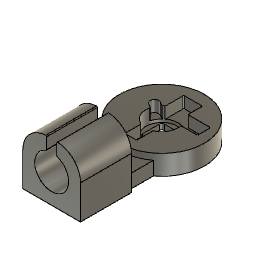
miniscope holder niko's version v13 (Autodesk Fusion 360 design; units mm, degrees)
Autodesk Fusion 360 part; units mm, degrees
sketch "Sketch1" plane through (0, 0, 0) normal (0, 1, 0) x (1, 0, 0)
  line L0 (0, 0) -> (0, -10)
  circle A0 centre (7, -10) radius 7 construction
  line L1 (0, 0) -> (8.5, 0)
  arc A1 (0, -10) -> (7, -17) centre (7, -10) ccw
  circle A2 centre (8.5, -8.5) radius 5 construction
  arc A3 (8.5, -3.5) -> (7, -13.2697) centre (8.5, -8.5) ccw
  line L2 (7, -13.2697) -> (7, -17)
  line L3 (8.5, 3.4063) -> (8.5, -43) construction
  arc A4 (10, -13.2697) -> (8.5, -3.5) centre (8.5, -8.5) ccw
  line L4 (10, -13.2697) -> (10, -17)
  line L5 (17, 0) -> (17, -10)
  arc A5 (10, -17) -> (17, -10) centre (10, -10) ccw
  line L6 (17, 0) -> (8.5, 0)
  dimension "d1" = 14
  dimension "d2" = 17
  dimension "d3" = 10
  dimension "d5" = 8.5
  dimension "d6" = 17
  dimension "d7" = 3
  constraint coincident L0.start L1.start
  constraint vertical L0
  constraint perpendicular L0 L1
  constraint coincident L0.end A0
  constraint coincident A0.centre A1.centre
  constraint vertical L1.end A2.centre
  constraint coincident A2 A3.start
  constraint coincident A2 A3.end
  constraint coincident A2.centre A3.centre
  constraint vertical L2
  constraint coincident A1.end L2.end
  constraint perpendicular L1 L3
  constraint vertical L1.end A3.start
  constraint symmetric L0.start L3 L5.start
  constraint symmetric L0.end L3 L5.end
  constraint symmetric L1.end L3 L6.end
  constraint symmetric A1.end L3 L4.end
  constraint symmetric A1 L3 A5
  constraint symmetric A3.start L3 A4.end
  constraint symmetric A3.end L3 A4.start
  constraint symmetric A3 L3 A4
  constraint coincident L1.end L3
  constraint horizontal L0.end A0.centre
  measures "d1" diameter of A0
  measures "d2" distance of L0 L5
  measures "d3" diameter of A2
  measures "d5" distance of A2.centre L6
  measures "d6" distance of L4.end L6
  measures "d7" distance of L2 L4
extrude "Extrude1" add sketch "Sketch1" along normal blind 15 makes body 1
sketch "Sketch2" plane through (0, 0, 0) normal (0, 0, 1) x (1, 0, 0)
  line L0 (17, 15) -> (0, 15)
  line L1 (8.5, 10.412) -> (8.5, 54) construction
  line L2 (1, 15) -> (1, 22.5)
  line L3 (16, 15) -> (16, 22.5)
  circle A0 centre (8.5, 32.5) radius 4.7
  line L4 (8.5, 32.5) -> (27, 32.5) construction
  line L5 (8.5, 32.5) -> (-9.7391, 43.0304) construction
  line L6 (8.5, 32.5) -> (17.9, 32.5) construction
  circle A1 centre (3.3471, 35.475) radius 1.25 construction
  circle A2 centre (8.5, 26.55) radius 1.25 construction
  circle A3 centre (13.6529, 35.475) radius 1.25 construction
  line L7 (5.75, 41.7) -> (11.25, 41.7)
  line L8 (17.95, 37.4) -> (17.95, 33.55)
  line L9 (6.75, 23.3) -> (10.25, 23.3)
  line L10 (5.75, 41.7) -> (5.75, 36.3115)
  line L11 (11.25, 41.7) -> (11.25, 37.4)
  line L12 (17.95, 37.4) -> (11.25, 37.4)
  line L13 (17.95, 33.55) -> (13.0812, 33.55)
  line L14 (6.75, 23.3) -> (6.75, 28.1379)
  line L15 (10.25, 23.3) -> (10.25, 28.1379)
  line L16 (13.2, 31.2992) -> (13.2, 33.7008) construction
  line L17 (9.7008, 37.2) -> (7.2992, 37.2) construction
  line L18 (3.8, 33.7008) -> (3.8, 31.2992) construction
  line L19 (7.2992, 27.8) -> (9.7008, 27.8) construction
  line L20 (13.6529, 35.475) -> (15.6, 35.475) construction
  arc A4 (3.9721, 36.5575) -> (2.7221, 34.3925) centre (3.3471, 35.475) ccw
  line L21 (3.9721, 36.5575) -> (5.2013, 35.8479)
  line L22 (2.7221, 34.3925) -> (3.9513, 33.6828)
  circle A5 centre (8.5, 32.5) radius 12.5
  line L23 (8.5, 20) -> (13, 20) construction
  line L24 (5.25, 35.75) -> (11.75, 35.75)
  line L25 (11.75, 35.75) -> (11.75, 29.25)
  line L26 (11.75, 29.25) -> (5.25, 29.25)
  line L27 (5.25, 29.25) -> (5.25, 35.75)
  line L28 (11.75, 35.75) -> (5.25, 29.25) construction
  dimension "d53" = 15
  dimension "d56" = 9.4
  dimension "d57" = 150
  dimension "d62" = 360
  dimension "d65" = 360
  dimension "d66" = 4.5
  dimension "d67" = 5.5
  dimension "d68" = 4.75
  dimension "d69" = 3.85
  dimension "d70" = 4.5
  dimension "d71" = 3.5
  dimension "d72" = 2.5
  dimension "d73" = 5
  dimension "d74" = 25
  dimension "d75" = 6.5
  constraint perpendicular L0 L1
  constraint coincident L0 L2.start
  constraint perpendicular L0 L2
  constraint coincident L0 L3.start
  constraint perpendicular L0 L3
  constraint symmetric L0.start L0.end L1
  constraint coincident A0.centre L4.start
  constraint perpendicular L1 L4
  constraint horizontal L6
  constraint coincident L5 A1.centre
  constraint tangent A0 A1
  constraint perpendicular L1 L7
  constraint horizontal L9
  constraint perpendicular L7 L10
  constraint perpendicular L7 L11
  constraint perpendicular L8 L12
  constraint perpendicular L8 L13
  constraint perpendicular L9 L14
  constraint perpendicular L9 L15
  constraint coincident A0 L10.end
  constraint coincident L11.end L12.end
  constraint coincident A0 L13.end
  constraint coincident A0 L14.end
  constraint coincident A0 L15.end
  constraint symmetric L1 L7.start L7.end
  constraint symmetric L1 L9.start L9.end
  constraint perpendicular L6 L16
  constraint tangent A0 L16
  constraint midpoint L6 L16
  constraint coincident A3.centre L20.start
  constraint horizontal L20
  constraint coincident A1 A4.start
  constraint coincident A1 A4.end
  constraint coincident A1.centre A4.centre
  constraint coincident A0 L21.end
  constraint coincident A0 L22.end
  constraint tangent A1 L22
  constraint tangent A1 L21
  constraint coincident A4.start L21.start
  constraint coincident A4.end L22.start
  constraint symmetric L5 L21 L22
  constraint parallel L21 L22
  constraint concentric A0 A5
  constraint coincident L3.end A5
  constraint coincident L2.end A5
  constraint coincident A5 L23.start
  constraint coincident L1 L23.start
  constraint perpendicular L1 L23
  constraint coincident L1 A0.centre
  constraint horizontal L24
  constraint perpendicular L24 L25
  constraint perpendicular L25 L26
  constraint perpendicular L24 L27
  constraint midpoint A0.centre L28
  constraint equal L26 L27
  measures "d53" distance of L2 L3
  measures "d56" diameter of A0
  measures "d57" angle of L5 L6
  measures "d66" distance of L7 L17
  measures "d67" distance of L7.start L7.end
  measures "d68" distance of L8 L16
  measures "d69" distance of L8.start L8.end
  measures "d70" distance of L9 L19
  measures "d71" distance of L9.start L9.end
  measures "d72" diameter of A1
  measures "d73" distance of L0 L23
  measures "d74" diameter of A5
  measures "d75" distance of L24.start L24.end
extrude "Extrude6" add sketch "Sketch2" along normal blind 4 contours L0 L2 L3 A5 bodies 1
extrude "Extrude7" add sketch "Sketch2" along normal blind 1.6 separate body contours A0 makes body 2
extrude "Extrude8" add sketch "Sketch2" along normal blind 2.5 contours A0 L7 L8 L10 L11 L12 L13 | A0 L9 L14 L15 | A0 A4 L21 L22 bodies 2
extrude "Extrude9" add sketch "Sketch2" along normal blind 5.85 contours A5 bodies 1 2
sketch "Sketch4" plane through (0, 0, 5.85) normal (0, 0, 1) x (-1, 0, 0)
  arc A0 (-3.9721, -36.5575) -> (-2.7221, -34.3925) centre (-3.3471, -35.475) ccw
  line L0 (-3.9721, -36.5575) -> (-5.2013, -35.8479)
  arc A1 (-5.75, -36.3115) -> (-5.2013, -35.8479) centre (-8.5, -32.5) ccw
  line L1 (-5.75, -36.3115) -> (-5.75, -41.7)
  line L2 (-5.75, -41.7) -> (-11.25, -41.7)
  line L3 (-11.25, -41.7) -> (-11.25, -37.4)
  line L4 (-11.25, -37.4) -> (-17.95, -37.4)
  line L5 (-17.95, -37.4) -> (-17.95, -33.55)
  line L6 (-17.95, -33.55) -> (-13.0812, -33.55)
  arc A2 (-10.25, -28.1379) -> (-13.0812, -33.55) centre (-8.5, -32.5) ccw
  line L7 (-10.25, -28.1379) -> (-10.25, -23.3)
  line L8 (-10.25, -23.3) -> (-6.75, -23.3)
  line L9 (-6.75, -23.3) -> (-6.75, -28.1379)
  arc A3 (-3.9513, -33.6828) -> (-6.75, -28.1379) centre (-8.5, -32.5) ccw
  line L10 (-3.9513, -33.6828) -> (-2.7221, -34.3925)
  circle A4 centre (-8.5, -32.5) radius 12.5
  circle A5 centre (-8.5, -32.5) radius 4.7
  line L11 (-8.5, -10.412) -> (-8.5, -54)
  line L12 (-11.75, -35.75) -> (-5.25, -29.25)
  line L13 (-2.5, -27.125) -> (-14.5, -27.125) construction
  line L14 (-14.5, -27.125) -> (-14.5, -37.875) construction
  line L15 (-14.5, -37.875) -> (-2.5, -37.875) construction
  line L16 (-2.5, -37.875) -> (-14.5, -27.125) construction
  line L17 (-5.75, -41.7) -> (-11.25, -41.7)
  line L18 (-17.95, -37.4) -> (-17.95, -33.55)
  line L19 (-6.75, -23.3) -> (-10.25, -23.3)
  line L20 (-2.5, -41.7) -> (-14.5, -41.7)
  line L21 (-14.5, -41.7) -> (-14.5, -37.875)
  line L22 (-17.95, -37.875) -> (-14.5, -37.875)
  line L23 (-17.95, -37.875) -> (-17.95, -24.3179)
  line L24 (-13.95, -23.3) -> (-2.5, -23.3)
  line L25 (-2.5, -37.875) -> (-2.5, -27.125) construction
  line L26 (-2.5, -41.7) -> (-2.5, -23.3)
  line L27 (-13.95, -23.3) -> (-13.95, -21.2507)
  line L28 (-1.5, -33) -> (2.8301, -30.5)
  line L29 (2.8301, -30.5) -> (-1.5, -28)
  line L30 (-1.5, -28) -> (-1.5, -33)
  line L31 (-0.8, -30.5) -> (-2.2, -30.5) construction
  line L32 (-8.5, -32.5) -> (-17.9, -32.5)
  line L33 (2.3301, -30.5) -> (-1.25, -32.567)
  line L34 (-1.25, -32.567) -> (-1.25, -28.433)
  line L35 (-1.25, -28.433) -> (2.3301, -30.5)
  dimension "d103" = 10.75
  dimension "d104" = 12
  dimension "d105" = 4
  dimension "d108" = 60
  dimension "d109" = 60
  dimension "d118" = 5
  dimension "d119" = 0.25
  dimension "d120" = 0.25
  dimension "d121" = 1
  dimension "d139" = 2
  constraint perpendicular L9 L13
  constraint perpendicular L13 L14
  constraint perpendicular L11 L15
  constraint midpoint L12 L16
  constraint perpendicular L14 L20
  constraint perpendicular L15 L21
  constraint perpendicular L21 L22
  constraint perpendicular L22 L23
  constraint perpendicular L13 L25
  constraint perpendicular L24 L26
  constraint coincident A4 L27.end
  constraint perpendicular L24 L27
  constraint coincident A4 L23.end
  constraint collinear L17 L20
  constraint collinear L19 L24
  constraint collinear L18 L23
  constraint coincident L15.end L16.start
  constraint collinear L25 L26
  constraint vertical L30
  constraint perpendicular L30 L31
  constraint midpoint L30 L31
  constraint parallel L28 L33
  constraint vertical L34
  constraint parallel L29 L35
  constraint symmetric L31 L33.end L34.end
  measures "d103" distance of L13.end L14.end
  measures "d104" distance of L13.start L13.end
  measures "d105" distance of L23 L27
  measures "d108" angle of L28 L29
  measures "d109" angle of L28 L30
  measures "d118" distance of L28.start L28.end
  measures "d119" distance of L28 L33
  measures "d120" distance of L30 L34
  measures "d121" distance of L25 L30
  measures "d139" distance of L31 L32
copy_body "Body->Comp1" bodies 1 removing the originals makes body 3 in component "base"
extrude "Extrude1'" add sketch "Sketch4" along normal blind 14 separate body contours A0 L26 | A0 L2 L8 A4 L11 L17 L19 L20 L24 L26 | L2 L5 A4 L11 L17 L18 L20 L21 L22 L23 | L8 A4 L11 L19 L24 L27 | L28 L29 L30 | L33 L34 L35 makes body 4 in component "lid"
extrude "Extrude2" cut 1 faces at (3.4069, 35.312, 2.5) along direction (0, 0, 1) blind 5.3 on bodies 3 bodies 4 in component "lid"
extrude "Extrude2'" [suppressed] in component "base"
extrude "Extrude3" cut sketch "Sketch4" along normal blind 5.25 contours L28 L29 L30 | L33 L34 L35 bodies 4 in component "lid"
fillet "Fillet2" [suppressed] in component "base"
extrude "Extrude4" add sketch "Sketch2" along normal blind 2 from surface at 19.85 contours A5 | A0 | A0 L7 L8 L10 L11 L12 L13 | A0 L9 L14 L15 | A0 A4 L21 L22 | L24 L25 L26 L27 bodies 4 in component "lid"
fillet "Fillet3" radius 0.25 13 edges at (6.75, 28.1379, 4.175) (3.9513, 33.6828, 4.175) (5.2013, 35.8479, 4.175) (5.75, 36.3115, 4.175) (11.25, 37.4, 4.175) (17.95, 37.4, 4.175) (17.95, 33.55, 4.175) (13.0812, 33.55, 4.175) (10.25, 28.1379, 4.175) (10.25, 23.3, 4.175) (6.75, 23.3, 4.175) (5.75, 41.7, 4.175) (11.25, 41.7, 4.175) on bodies 3 in component "base"
fillet "Fillet3" radius 0.25 4 edges at (7, 7.5, 17) (7, 7.5, 13.2697) (10, 7.5, 17) (10, 7.5, 13.2697) on bodies 3 in component "base"
fillet "Fillet4" radius 0.75 4 edges at (5.25, 35.75, 0.8) (11.75, 35.75, 0.8) (11.75, 29.25, 0.8) (5.25, 29.25, 0.8) on bodies 3 in component "base"
fillet "Fillet1" radius 0.25 9 edges at (2.5, 34.5558, 6.825) (2.5, 36.3942, 6.825) (2.5, 41.7, 12.85) (14.5, 41.7, 12.85) (14.5, 37.875, 12.85) (17.95, 37.875, 12.85) (17.95, 24.3179, 12.85) (13.95, 23.3, 12.85) (2.5, 23.3, 12.85) on bodies 4 in component "lid"
component "lid" placed x (1, 0, 0) y (0, 1, 0) z (0, 0, 1) at (0, 0, 0)
component "base" placed x (1, 0, 0) y (0, 1, 0) z (0, 0, 1) at (0, 0, 0)
